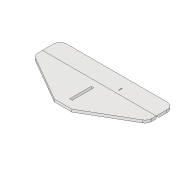
# Autodesk Inventor part: horizontal_stabilizer
Saved by Autodesk Inventor 2019 (Build 230136000, 136)
## iProperties
Created: 2022-03-20
Part Number: horizontal_stabilizer
Material: Foam board
Document SubType Name: Modeling
Designer: solyo
Density: 0.096049 g/cm^3
Appearance: Foam
Mass: 8.16341 g
Surface Area: 399.482 cm^2
Volume: 84.9922 cm^3
Author: solyo
Autodesk Inventor part; units mm, degrees
ref_plane "YZ Plane" through (0, 0, 0) normal (1, 0, 0) x (0, 1, 0)
ref_plane "XZ Plane" through (0, 0, 0) normal (0, 1, 0) x (-1, 0, 0)
sketch "Sketch1" plane through (0, 0, 0) normal (0, 1, 0) x (-1, 0, 0)
  line L0 (17, 0) -> (-17, 0)
  line L1 (-17, 0) -> (-110, -54)
  line L2 (-110, -54) -> (-110, -104)
  line L3 (-110, -104) -> (110, -104)
  line L4 (110, -104) -> (110, -54)
  line L5 (110, -54) -> (17, 0)
  point P0 (0, 0)
  dimension "d0" = 220
  dimension "d1" = 104
  dimension "d4" = 34
  dimension "d5" = 17
  dimension "d8" = 50
  constraints: 12 end point, 3 perpendicular, 2 equal length, 1 horizontal, 1 midpoint
  measures "d0" distance of L2.end L3.end
  measures "d1" distance between parallel lines of L0 L3
  measures "d4" distance of L0.start L0.end
  measures "d5" distance of L0.end point (0, 0)
  measures "d8" distance of L3.end L4.end
extrude "Extrusion1" add sketch "Sketch1" along normal blind 5
fillet "Fillet1" radius 13 4 edges at (-110, 2.5, -104) (110, 2.5, -104) (110, 2.5, -54) (-110, 2.5, -54)
sketch "Sketch2" plane through (0, 5, 0) normal (0, 1, 0) x (1, 0, 0)
  line L0 (-2.5, 57) -> (2.5, 57)
  line L1 (2.5, 57) -> (2.5, 15)
  line L2 (2.5, 15) -> (-2.5, 15)
  line L3 (-2.5, 15) -> (-2.5, 57)
  line L4 (-17, 0) -> (17, 0) projected
  line L5 (0, 0) -> (0, 5.9435) construction
  line L6 (30, 83) -> (31.5, 83)
  line L7 (31.5, 83) -> (31.5, 77)
  line L8 (31.5, 77) -> (30, 77)
  line L9 (30, 77) -> (30, 83)
  line L10 (110, 61.4842) -> (110, 91) projected
  line L11 (97, 104) -> (-97, 104) projected
  point P0 (0, 0)
  point P1 (0, 15)
  dimension "d12" = 5
  dimension "d13" = 42
  dimension "d14" = 15
  dimension "d28" = 1.5
  dimension "d29" = 78.5
  dimension "d30" = 21
  dimension "d31" = 6
  constraints: 18 end point, 4 parallel, 2 horizontal, 2 midpoint, 2 perpendicular, 1 vertical, 1 vertical alignment
  measures "d12" distance of L1.end L2.end
  measures "d13" distance of L0.end L1.end
  measures "d14" distance between parallel lines of L4 L2
  measures "d28" distance between parallel lines of L7 L9
  measures "d29" distance between parallel lines of L10 L7
  measures "d30" distance between parallel lines of L11 L6
  measures "d31" distance of L6.end L7.end
extrude "Extrusion2" cut sketch "Sketch2" against normal through all
sketch "Sketch3" plane through (110, 0, -61.4842) normal (1, 0, 0) x (0, 0, -1)
  line L0 (42.5158, 0) -> (42.5158, 5) projected
  line L1 (0, 5) -> (29.5158, 5) projected
  line L2 (29.5158, 0) -> (0, 0) projected
  line L3 (29.5158, 5) -> (0, 5) projected
  line L4 (8.5158, 0) -> (8.5158, 5)
  line L5 (8.5158, 0) -> (13.5158, 0)
  line L6 (0, 0) -> (29.5158, 0) projected
  line L7 (8.5158, 5) -> (13.5158, 0)
  point P0 (-61.4842, 0)
  dimension "d26" = 45
  dimension "d27" = 34
  constraints: 6 end point, 3 point on line
  measures "d26" angle of L2 L7
  measures "d27" distance between parallel lines of L0 L4
extrude "Extrusion3" cut sketch "Sketch3" against normal through all
ref_plane "Work Plane1" through (110, 0, -70) normal (0, 0, -1) x (-1, 0, 0)
split body "Split1" result two bodies by plane through (110, 0, -70) normal (0, 0, -1) first body at (-59, 4.5, -83.6667)
equation "\"d5\" = 0.5 * d4"
equation "\"d9\" = Thickness"
equation "\"d12\" = Thickness"
equation "\"d23\" = Thickness"
equation "\"Thickness\" = 5"
